Autodesk Inventor part; units mm, degrees
(part 2 of 2)
  line L1063 (-236, -22.5) -> (-236, -25.5)
  line L1064 (-159, -34.5) -> (-156, -34.5)
  line L1065 (-156, -34.5) -> (-156, -25.5)
  line L1066 (-156, -25.5) -> (-159, -25.5)
  line L1067 (-159, -25.5) -> (-159, -34.5)
  line L1068 (-172, -25.5) -> (-172, -22.5)
  line L1069 (-172, -22.5) -> (-182, -22.5)
  line L1070 (-182, -25.5) -> (-172, -25.5)
  line L1071 (-182, -22.5) -> (-182, -25.5)
  line L1072 (-288, -15) -> (-288, -24)
  line L1073 (-288, -24) -> (-291, -24)
  line L1074 (-291, -15) -> (-288, -15)
  line L1075 (-288, -24) -> (-291, -24)
  line L1076 (-251.5, -55) -> (-241.5, -55)
  line L1077 (-241.5, -58) -> (-251.5, -58)
  line L1078 (-251.5, -55) -> (-241.5, -55)
  line L1079 (-241.5, -58) -> (-251.5, -58)
  line L1080 (-251.5, -58) -> (-241.5, -58)
  line L1081 (-241.5, -55) -> (-241.5, -58)
  line L1082 (-241.5, -55) -> (-241.5, -58)
  line L1083 (-241.5, -58) -> (-241.5, -55)
  line L1084 (-251.5, -58) -> (-251.5, -55)
  line L1085 (-251.5, -55) -> (-251.5, -58)
  line L1086 (-251.5, -58) -> (-251.5, -55)
  line L1087 (-259, -55) -> (-259, -58)
  line L1088 (-259, -52) -> (-259, -55)
  line L1089 (-259, -58) -> (-262, -58)
  line L1090 (-262, -58) -> (-262, -52)
  line L1091 (-262, -52) -> (-259, -52)
  line L1092 (-176.5, -55) -> (-176.5, -58)
  line L1093 (-176.5, -58) -> (-166.5, -58)
  line L1094 (-166.5, -58) -> (-166.5, -55)
  line L1095 (-166.5, -55) -> (-176.5, -55)
  line L1096 (-159, -52) -> (-159, -58)
  line L1097 (-156, -55) -> (-156, -52)
  line L1098 (-156, -52) -> (-159, -52)
  line L1099 (-156, -58) -> (-156, -55)
  line L1100 (-159, -58) -> (-156, -58)
  line L1101 (-209, -6.875) -> (-191, -6.875)
  line L1102 (-191, -6.875) -> (-191, -9.875)
  line L1103 (-191, -9.875) -> (-209, -9.875)
  circle A51 centre (-189, 8.0625) radius 1.5
  line L1104 (-194.5, 25) -> (-197.5, 25)
  line L1105 (-197.5, 25) -> (-197.5, 35)
  line L1106 (-197.5, 35) -> (-194.5, 35)
  line L1107 (-194.5, 35) -> (-194.5, 25)
  line L1108 (-288, -89) -> (-291, -89)
  line L1109 (-291, -24) -> (-291, -15)
  line L1110 (-291, 15) -> (-291, 24)
  line L1111 (-291, 24) -> (-288, 24)
  line L1112 (-288, 15) -> (-291, 15)
  line L1113 (-288, 24) -> (-288, 15)
  line L1114 (-127, -24) -> (-130, -24)
  line L1115 (-130, -15) -> (-127, -15)
  line L1116 (-130, 24) -> (-130, 15)
  line L1117 (-127, 24) -> (-130, 24)
  line L1118 (-127, 15) -> (-127, 24)
  line L1119 (-127, 15) -> (-130, 15)
  line L1120 (-130, -24) -> (-130, -15)
  line L1121 (-127, -15) -> (-127, -24)
  line L1122 (-127, -24) -> (-130, -24)
  line L1123 (-130, -89) -> (-127, -89)
  line L1124 (-294, -95) -> (-124, -95)
  line L1125 (-124, -95) -> (-124, 95)
  line L1126 (-121, -15) -> (-121, 15)
  circle A52 centre (18.75, 15.75) radius 1.5
  circle A53 centre (-18.75, 15.75) radius 1.5
  circle A54 centre (-18.75, 53.25) radius 1.5
  circle A55 centre (18.75, 53.25) radius 1.5
  circle A56 centre (18.75, -53.25) radius 1.5
  circle A57 centre (-18.75, -53.25) radius 1.5
  circle A58 centre (-18.75, -15.75) radius 1.5
  circle A59 centre (18.75, -15.75) radius 1.5
  point P0 (-405.4327, -62.749)
  point P1 (-408.4327, -62.749)
  point P2 (-102, 54)
  point P3 (-97, 59)
  point P4 (-92, 82)
  point P5 (-97, 87)
  point P6 (-112, 87)
  point P7 (-117, 82)
  point P8 (-112, 59)
  point P9 (-107, 54)
  point P10 (-102, 18)
  point P11 (-97, 23)
  point P12 (-97, 46)
  point P13 (-97, 51)
  point P14 (-112, 51)
  point P15 (-117, 46)
  point P16 (-112, 46)
  point P17 (-112, 23)
  point P18 (-107, 18)
  point P19 (-112, -30.5)
  point P20 (-112, -53.5)
  point P21 (-107, -58.5)
  point P22 (-102, -58.5)
  point P23 (-97, -53.5)
  point P24 (-97, -30.5)
  point P25 (-92, -30.5)
  point P26 (-97, -25.5)
  point P27 (-112, -25.5)
  point P28 (-117, -30.5)
  point P29 (-112, -89.5)
  point P30 (-107, -94.5)
  point P31 (-102, -94.5)
  point P32 (-97, -89.5)
  point P33 (-97, -66.5)
  point P34 (-92, -66.5)
  point P35 (-97, -61.5)
  point P36 (-112, -61.5)
  point P37 (-117, -66.5)
  point P38 (-112, -66.5)
  point P39 (198, -18)
  point P40 (168, 15)
  point P41 (168, -15)
  point P42 (-124, 95)
  point P43 (-130, -89)
  point P44 (-127, -89)
  point P45 (-288, -89)
  point P46 (-127, 15)
  point P47 (-291, 89)
  point P48 (-127, 89)
  point P49 (-130, 80)
  point P50 (-291, -15)
  point P51 (-130, -15)
  point P52 (15, 111.5)
  point P53 (-85, -15)
  point P54 (-5.25, -2)
  point P55 (-5.25, 2)
  point P56 (82, 15)
  point P57 (-79, -15)
  point P58 (-82, -15)
  point P59 (82, 80)
  point P60 (79, 89)
  point P61 (82, -24)
  point P62 (79, -15)
  point P63 (-79, 89)
  point P64 (-79, 80)
  point P65 (55.9446, -123.4202)
  point P66 (55.9446, -104.4202)
  point P67 (72.1946, -113.9202)
  point P68 (61.4446, -113.9202)
  point P69 (-335.9327, -61.249)
  point P70 (-361.9327, -61.249)
  point P71 (-348.9327, -61.249)
  point P72 (-342.4327, -62.749)
  point P73 (-405.4327, -59.749)
  point P74 (-374.9327, -61.249)
  point P75 (-408.4327, -61.249)
  point P76 (-405.4327, -9.749)
  point P77 (-374.9327, -8.249)
  point P78 (-361.9327, -8.249)
  point P79 (-348.9327, -8.249)
  point P80 (-335.9327, -8.249)
  point P81 (-312.9327, 8.1476)
  point P82 (-335.9327, 8.1476)
  point P83 (-322.9327, 8.1476)
  point P84 (-361.9327, 8.1476)
  point P85 (-348.9327, 8.1476)
  point P86 (-387.9327, 8.1476)
  point P87 (-374.9327, 8.1476)
  point P88 (-397.9327, 8.1476)
  point P89 (-408.4327, 11.1476)
  point P90 (-368.4327, -6.749)
  point P91 (324.5, 92)
  point P92 (207, -52)
  point P93 (208.5, 58)
  point P94 (249, 90.5)
  point P95 (320, 90.5)
  point P96 (258, 90.5)
  point P97 (329, 90.5)
  point P98 (208.5, -46)
  point P99 (208.5, 46)
  point P100 (208.5, -58)
  point P101 (296.5, 128)
  point P102 (279, 126.5)
  point P103 (284, 126.5)
  point P104 (294, 126.5)
  point P105 (299, 126.5)
  point P106 (35.5, -92)
  point P107 (82, 84.5)
  point P108 (80.5, 89)
  point P109 (80.5, 80)
  point P110 (80.5, 58)
  point P111 (80.5, 24)
  point P112 (80.5, 46)
  point P113 (80.5, -24)
  point P114 (80.5, -46)
  point P115 (80.5, -58)
  point P116 (80.5, -80)
  point P117 (80.5, -89)
  point P118 (35.5, 111.5)
  point P119 (35.5, 92)
  point P120 (35.5, 89)
  point P121 (-35.5, 92)
  point P122 (23, 108.5)
  point P123 (-7.5, 128)
  point P124 (5, 126.5)
  point P125 (-5, 126.5)
  point P126 (-10, 126.5)
  point P127 (10, 126.5)
  point P128 (57.5, -85.5)
  point P129 (121, 0)
  point P130 (58.0916, -22)
  point P131 (37, -24)
  point P132 (56, -24)
  point P133 (57.5, -70.5)
  point P134 (58.0916, -26)
  point P135 (32, -25.5)
  point P136 (52.5, 30)
  point P137 (14.5, 30)
  point P138 (49.5, 30)
  point P139 (-11.5, 30)
  point P140 (11.5, 30)
  point P141 (-49.5, 30)
  point P142 (-14.5, 30)
  point P143 (-52.5, 30)
  point P144 (-5.25, 0)
  point P145 (-9.25, 0)
  point P146 (59, 78)
  point P147 (59, -78)
  point P148 (40, -90.5)
  point P149 (-31, -90.5)
  point P150 (31, -90.5)
  point P151 (-40, -90.5)
  point P152 (-37, 84)
  point P153 (37, 84)
  point P154 (-59, 78)
  point P155 (-166.5, -3.5)
  point P156 (-159, -5)
  point P157 (-128.5, -89)
  point P158 (-128.5, -24)
  point P159 (-128.5, 24)
  point P160 (-128.5, 89)
  point P161 (-288, -84.5)
  point P162 (-209, -95)
  point P163 (-261.5, 30)
  point P164 (-223.5, 30)
  point P165 (-197.5, 30)
  point P166 (-159.5, 30)
  point P167 (-194.5, 30)
  point P168 (-241, 85.5)
  point P169 (-189, 107)
  point P170 (-165.5, 107)
  point P171 (-183, 107)
  point P172 (-156.5, 107)
  point P173 (-260.5, -34.5)
  point P174 (-260.5, -52)
  point P175 (-260.5, -8)
  point P176 (-260.5, -25.5)
  point P177 (-251.5, -56.5)
  point P178 (-176.5, -56.5)
  point P179 (-241.5, -56.5)
  point P180 (-166.5, -56.5)
  point P181 (-262, -55)
  dimension "d226" = 18
  dimension "d228" = 5
  dimension "d231" = 16
  dimension "d232" = 9
  dimension "d233" = 16
  dimension "d234" = 35
  dimension "d235" = 3
  dimension "d236" = 10
  dimension "d237" = 5
  dimension "d238" = 5
  dimension "d239" = 5
  dimension "d240" = 35
  dimension "d242" = 37
  dimension "d243" = 12
  dimension "d244" = 31
  dimension "d245" = 12.5
  dimension "d246" = 35
  dimension "d247" = 3
  dimension "d248" = 70
  dimension "d249" = 36
  dimension "d250" = 30
  dimension "d251" = 5
  dimension "d252" = 3
  dimension "d253" = 9
  dimension "d254" = 3
  dimension "d255" = 12
  dimension "d256" = 3
  dimension "d257" = 25
  dimension "d258" = 5
  dimension "d259" = 9
  dimension "d260" = 5
  dimension "d261" = 3
  dimension "d262" = 25
  dimension "d263" = 10
  dimension "d264" = 10
  dimension "d265" = 10
  dimension "d266" = 3
  dimension "d267" = 3
  dimension "d268" = 10
  dimension "d269" = 5
  dimension "d270" = 25
  dimension "d271" = 9
  dimension "d272" = 5
  dimension "d273" = 17.5
  dimension "d274" = 6
  dimension "d275" = 3
  dimension "d277" = 11
  dimension "d279" = 3
  dimension "d280" = 19
  dimension "d281" = 3
  dimension "d282" = 10.75
  dimension "d283" = 18.75
  dimension "d284" = 15
  dimension "d285" = 10
  dimension "d286" = 15
  dimension "d287" = 25
  dimension "d288" = 3
  dimension "d289" = 30
  dimension "d290" = 80
  dimension "d291" = 80
  dimension "d292" = 70
  dimension "d294" = 30
  dimension "d295" = 70
  dimension "d298" = 10
  constraints: 2254 end point, 117 midpoint, 60 centre point, 32 point on circle, 5 perpendicular, 2 parallel
  measures "d226" diameter of A22
  measures "d228" distance of L181.start L181.end
  measures "d231" distance of L522.start L522.end
  measures "d232" distance of L520.start L520.end
  measures "d233" distance of L518.start L518.end
  measures "d234" distance of L720.start L720.end
  measures "d235" distance of L519.start L519.end
  measures "d236" distance of L179.start L179.end
  measures "d237" distance of L177.start L177.end
  measures "d238" distance of L175.start L175.end
  measures "d239" distance of L183.start L183.end
  measures "d240" distance of L164.start L164.end
  measures "d242" distance of L116.start L116.end
  measures "d243" distance of L118.start L118.end
  measures "d244" distance of L120.start L120.end
  measures "d245" diameter of A20
  measures "d246" distance of L115.start L115.end
  measures "d247" distance of L119.start L119.end
  measures "d248" distance of L480.start L480.end
  measures "d249" distance of L481.start L481.end
  measures "d250" distance of L482.start L482.end
  measures "d251" distance of L82.start L82.end
  measures "d252" distance of L83.start L83.end
  measures "d253" distance of L138.start L138.end
  measures "d254" distance of L139.start L139.end
  measures "d255" distance of L65.start L65.end
  measures "d256" distance of L64.start L64.end
  measures "d257" distance of L497.start L497.end
  measures "d258" distance of L498.start L498.end
  measures "d259" distance of L506.start L506.end
  measures "d260" distance of L504.start L504.end
  measures "d261" distance of L505.start L505.end
  measures "d262" distance of L537.start L537.end
  measures "d263" distance of L534.start L534.end
  measures "d264" distance of L532.start L532.end
  measures "d265" distance of L536.start L536.end
  measures "d266" distance of L535.start L535.end
  measures "d267" distance of L207.start L207.end
  measures "d268" diameter of A24
  measures "d269" distance of L206.start L206.end
  measures "d270" distance of L224.start L224.end
  measures "d271" distance of L227.start L227.end
  measures "d272" distance of L225.start L225.end
  measures "d273" distance of L229.start L229.end
  measures "d274" distance of L231.start L231.end
  measures "d275" distance of L759.start L759.end
  measures "d277" distance of L441.start L441.end
  measures "d279" distance from line of L234 point (55.945, -104.42)
  measures "d280" distance of L440.start L440.end
  measures "d281" distance from line of L229 point (55.945, -123.42)
  measures "d282" distance of point (72.195, -113.92) point (61.445, -113.92)
  measures "d283" distance from line of L224 L439.end
  measures "d284" distance of L248.start L248.end
  measures "d285" distance of L250.start L250.end
  measures "d286" distance of L252.start L252.end
  measures "d287" distance of L259.start L259.end
  measures "d288" distance of L249.start L249.end
  measures "d289" distance of L703.start L703.end
  measures "d290" distance of L485.start L485.end
  measures "d291" distance of L487.start L487.end
  measures "d292" distance of L486.start L486.end
  measures "d294" distance of L707.start L707.end
  measures "d295" distance of L474.start L474.end
  measures "d298" distance of L274.start L274.end
extrude "Extrusión1" add sketch "Boceto1" along normal blind 3
